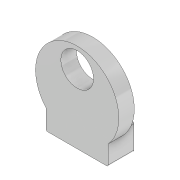
# Autodesk Inventor part: ZWO-EFW-Mini
Saved by Autodesk Inventor 2021 (Build 250183000, 183)
## iProperties
Created: 2022-11-28
Part Number: ZWO-EFW-Mini
Material: Generic
Document SubType Name: Modeling
Designer: nvladi
Density: 1 g/cm^3
Appearance: Anodized - Light Gray
Author: nvladi
Autodesk Inventor part; units mm, degrees
ref_plane "YZ Plane" through (0, 0, 0) normal (1, 0, 0) x (0, 1, 0)
ref_plane "XZ Plane" through (0, 0, 0) normal (0, 1, 0) x (-1, 0, 0)
ref_plane "XY Plane" through (0, 0, 0) normal (0, 0, 1) x (1, 0, 0)
sketch "Sketch1" plane through (0, 0, 0) normal (0, 0, 1) x (1, 0, 0)
  circle A0 centre (0, 0) radius 53.5
  line L0 (38, -61) -> (-38, -61)
  line L1 (-40, -59) -> (-40, -35.5282)
  line L2 (40, -61) -> (-40, 61) construction
  line L3 (-40, -61) -> (40, 61) construction
  circle A1 centre (0, 27.5) radius 21
  line L4 (40, -35.5282) -> (40, -59)
  arc A2 (-40, -59) -> (-38, -61) centre (-38, -59) ccw
  arc A3 (38, -61) -> (40, -59) centre (38, -59) ccw
  dimension "d0" = 107
  dimension "d3" = 42
  dimension "d4" = 27.5
  dimension "d5" = 61
  dimension "d7" = 80
  dimension "d8" = 2
  constraints: 10 end point, 6 point on circle, 4 centre point, 4 point on line, 4 tangent, 2 midpoint, 1 coincident, 1 equal radius, 1 horizontal, 1 parallel, 1 perpendicular
  measures "d0" diameter of A0
  measures "d3" diameter of A1
  measures "d4" distance of point (0, 0) A1.centre
  measures "d5" distance from line of point (0, 0) L0
  measures "d7" distance between parallel lines of L4 L1
  measures "d8" radius of A2
extrude "Extrusion1" add sketch "Sketch1" along normal blind 20
sketch "Sketch2" plane through (0, 0, 20) normal (0, 0, 1) x (1, 0, 0)
  line L0 (38, -61) -> (-38, -61)
  line L1 (-40, -59) -> (-40, -29.5)
  line L2 (-38, -27.5) -> (38, -27.5)
  line L3 (40, -29.5) -> (40, -59)
  arc A0 (-38, -27.5) -> (-40, -29.5) centre (-38, -29.5) ccw
  arc A1 (40, -29.5) -> (38, -27.5) centre (38, -29.5) ccw
  arc A2 (38, -61) -> (40, -59) centre (38, -59) ccw
  arc A3 (-40, -59) -> (-38, -61) centre (-38, -59) ccw
  point P0 (0, 0)
  point P1 (-40, -27.5)
  point P2 (-40, -61)
  point P3 (40, -27.5)
  dimension "d11" = 80
  dimension "d12" = 33.5
  dimension "d13" = 2
  constraints: 8 end point, 8 point on circle, 8 tangent, 6 point on line, 4 centre point, 3 equal radius, 2 parallel, 1 horizontal, 1 perpendicular
  measures "d11" distance of point (-40, -27.5) point (40, -27.5)
  measures "d12" distance of point (-40, -61) point (-40, -27.5)
  measures "d13" radius of A0
extrude "Extrusion2" add sketch "Sketch2" along normal blind 13
body "Solid1"
